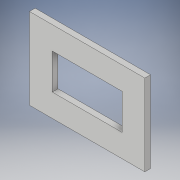
# Autodesk Inventor part: SmartServoHolderClaw
Saved by Autodesk Inventor 2017 (Build 210142000, 142)
## iProperties
Created: 2017-09-30
Part Number: SmartServoHolderClaw
Material: Generic
Document SubType Name: Modeling
Designer: User
Density: 1 g/cm^3
Appearance: Default
Author: User
Autodesk Inventor part; units mm, degrees
ref_plane "YZ Plane" through (0, 0, 0) normal (1, 0, 0) x (0, 1, 0)
ref_plane "XZ Plane" through (0, 0, 0) normal (0, 1, 0) x (-1, 0, 0)
ref_plane "XY Plane" through (0, 0, 0) normal (0, 0, 1) x (1, 0, 0)
sketch "Sketch1" plane through (0, 0, 0) normal (0, 0, 1) x (1, 0, 0)
  line L0 (0, 0) -> (0, 45.212)
  line L1 (0, 45.212) -> (64.2112, 45.212)
  line L2 (64.2112, 45.212) -> (64.2112, 0)
  line L3 (64.2112, 0) -> (0, 0)
  line L4 (12.7, 32.512) -> (51.5112, 32.512)
  line L5 (51.5112, 32.512) -> (51.5112, 12.7)
  line L6 (51.5112, 12.7) -> (12.7, 12.7)
  line L7 (12.7, 12.7) -> (12.7, 32.512)
  dimension "d0" = 45.212
  dimension "d1" = 64.2112
  dimension "d4" = 38.8112
  dimension "d5" = 19.812
  constraints: 16 end point, 4 perpendicular, 2 parallel, 1 horizontal, 1 vertical
  measures "d0" distance of L0.start L0.end
  measures "d1" distance of L0.end L1.end
  measures "d4" distance of L5.end L6.end
  measures "d5" distance of L4.end L5.end
extrude "Extrusion1" add sketch "Sketch1" along normal blind 3.175
body "Solid1"
